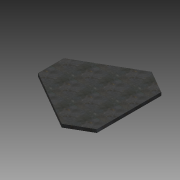
# Autodesk Inventor part: Platform
Saved by Autodesk Inventor 2015 (Build 190159000, 159)
## iProperties
Created: 2016-02-02
Part Number: Platform
Material: Steel
Document SubType Name: Modeling
Designer: tuttlem
Mass: 32237.8 g
Surface Area: 4761.07 cm^2
Volume: 4106.72 cm^3
Density: 7.85 g/cm^3
Appearance: Plate
Author: tuttlem
Autodesk Inventor part; units mm, degrees
ref_plane "YZ Plane" through (0, 0, 0) normal (1, 0, 0) x (0, 1, 0)
ref_plane "XZ Plane" through (0, 0, 0) normal (0, 1, 0) x (-1, 0, 0)
ref_plane "XY Plane" through (0, 0, 0) normal (0, 0, 1) x (1, 0, 0)
sketch "Sketch1" plane through (0, 0, 0) normal (0, 1, 0) x (-1, 0, 0)
  line L0 (613.6799, 122.9576) -> (173.739, 376.9576)
  line L1 (173.739, -334.2424) -> (613.6799, -80.2424)
  line L2 (613.6799, 122.9576) -> (613.6799, -80.2424)
  line L3 (173.739, 376.9576) -> (-2.2373, 275.3576)
  line L4 (173.739, -334.2424) -> (-2.2373, -232.6424)
  line L5 (-2.2373, 275.3576) -> (-2.2373, -232.6424)
  dimension "d0" = 203.2
  dimension "d6" = 508
  constraints: 12 end point, 2 parallel, 2 vertical, 2 other
  measures "d0" distance of L0.start L1.end
  measures "d6" distance of L0.start L0.end
extrude "Extrusion1" add sketch "Sketch1" along normal blind 25.4
body "Solid1"
